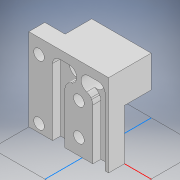
# Autodesk Inventor part: 000.012.001 - Основание
Saved by Autodesk Inventor 2022 (Build 260153000, 153)
## iProperties
Created: 2023-04-23
Part Number: 000.012.001 - Основание
Material: Типовые
Document SubType Name: Modeling
Designer: Иван Петров
Density: 1 g/cm^3
Appearance: По умолчанию
Author: Иван Петров
Autodesk Inventor part; units mm, degrees
ref_plane "YZ Plane" through (0, 0, 0) normal (1, 0, 0) x (0, 1, 0)
ref_plane "XZ Plane" through (0, 0, 0) normal (0, 1, 0) x (-1, 0, 0)
ref_plane "XY Plane" through (0, 0, 0) normal (0, 0, 1) x (1, 0, 0)
sketch "Эскиз1" plane through (0, 0, 0) normal (0, 0, 1) x (1, 0, 0)
  line L0 (-10, -10.5115) -> (10, -10.5115)
  line L1 (10, -10.5115) -> (10, 10.5115)
  line L2 (10, 10.5115) -> (-10, 10.5115)
  line L3 (-10, 10.5115) -> (-10, -10.5115)
  line L4 (-10, -10.5115) -> (10, 10.5115) construction
  line L5 (10, -10.5115) -> (-10, 10.5115) construction
  point P0 (0, 0)
  dimension "d0" = 20
  dimension "d1" = 21.023
  constraints: 12 end point, 2 midpoint, 2 parallel, 1 horizontal, 1 perpendicular
  measures "d0" distance of L2.end L1.end
  measures "d1" distance of L1.end L0.end
extrude "Выдавливание1" add sketch "Эскиз1" along normal blind 6
sketch "Эскиз2" plane through (0, 0, 6) normal (0, 0, 1) x (1, 0, 0)
  circle A0 centre (2.5, 4.5115) radius 2.85 projected
  circle A1 centre (-4.85, 4.5115) radius 2.85 projected
  point P0 (0, 0)
extrude "Выдавливание2" cut sketch "Эскиз2" against normal blind 6
move faces "Перенос1" translate (-10, 0, 0) faces at (-10, 3.5038, 2)
move faces "Перенос2" translate (0, -10, 0) faces at (-10, -10.5115, 2)
sketch "Эскиз4" plane through (0, 0, 0) normal (0, 0, -1) x (-1, 0, 0)
  line L0 (8.6, 0.7615) -> (-3.85, 0.7615) projected
  arc A0 (8.6, 0.7615) -> (9.1, 1.2615) centre (8.6, 1.2615) ccw projected
  line L1 (9.1, 7.7615) -> (9.1, 1.2615) projected
  line L2 (-3.85, 8.2615) -> (8.6, 8.2615) projected
  arc A1 (9.1, 7.7615) -> (8.6, 8.2615) centre (8.6, 7.7615) ccw projected
  line L3 (-6.75, 5.6615) -> (-3.85, 8.2615) projected
  line L4 (-6.75, 3.3615) -> (-6.75, 5.6615) projected
  line L5 (-3.85, 0.7615) -> (-6.75, 3.3615) projected
  line L6 (-10, 10.5115) -> (20, 10.5115) projected
  line L7 (-10, 10.5115) -> (12.35, 10.5115)
  line L8 (12.35, 10.5115) -> (12.35, -1.4885)
  line L9 (12.35, -1.4885) -> (-10, -1.4885)
  line L10 (-10, -1.4885) -> (-10, 10.5115)
  point P0 (0, 0)
  dimension "d19" = 2.25
  dimension "d20" = 2.25
  dimension "d21" = 3.25
  dimension "d23" = 3.25
  constraints: 8 end point, 2 parallel, 1 horizontal, 1 perpendicular
  measures "d19" distance between parallel lines of L6 L2
  measures "d20" distance between parallel lines of L0 L9
  measures "d21" distance between parallel lines of L10 L4
  measures "d23" distance between parallel lines of L8 L1
extrude "Выдавливание4" add sketch "Эскиз4" along normal blind 10
offset faces "Размер1" outward -0.5 faces at (-0.3, 8.2615, -3.3333) (-8.9665, 8.1016, -6.6667) (-9.1, 5.5948, -3.3333) (5.7833, 6.5282, -3.3333) (6.75, 4.1282, -3.3333) (4.8167, 1.6282, -3.3333) (-4.45, 0.7615, -3.3333) (-8.7474, 0.7837, -6.6667)
sketch "Эскиз5" plane through (0, 0, 0) normal (0, 0, -1) x (-1, 0, 0)
  circle A0 centre (16.175, 4.9639) radius 2
  line L0 (12.35, 10.5115) -> (20, 10.5115) projected
  point P0 (0, 0)
  point P1 (16.175, 10.5115)
  dimension "d27" = 4
  constraints: 1 centre point, 1 midpoint, 1 vertical alignment
  measures "d27" diameter of A0
extrude "Выдавливание5" cut sketch "Эскиз5" against normal blind 10
sketch "Эскиз6" plane through (0, 0, 6) normal (0, 0, 1) x (1, 0, 0)
  circle A0 centre (-16.175, -17.4699) radius 2
  circle A1 centre (-16.175, 4.9639) radius 2 projected
  circle A2 centre (-1.1985, -0.3999) radius 2
  point P0 (0, 0)
  dimension "d30" = 4
  dimension "d31" = 4
  constraints: 2 centre point, 1 vertical alignment
  measures "d30" diameter of A0
  measures "d31" diameter of A2
extrude "Выдавливание6" cut sketch "Эскиз6" against normal blind 6.5 contours A0
sketch "Эскиз7" plane through (0, 0, 6) normal (0, 0, 1) x (1, 0, 0)
  circle A0 centre (-4.85, 4.5115) radius 2.85 projected
  line L0 (-4.85, 7.3615) -> (-11.0596, 7.3615)
  line L1 (-11.0596, 7.3615) -> (-11.0596, -20.5115)
  line L2 (-20, -20.5115) -> (10, -20.5115) projected
  line L3 (-5, 1.6655) -> (-6.4302, -0.5077)
  line L4 (-6.4302, -0.5077) -> (-6.4302, -20.5115)
  line L5 (10, 10.5115) -> (-20, 10.5115) projected
  line L6 (-1.175, 10.5115) -> (-1.175, 2.4545) construction
  circle A1 centre (2.5, 4.5115) radius 2.85 projected
  line L7 (-4.85, 4.5115) -> (-4.85, 5.527) construction
  line L8 (2.5, 4.5115) -> (2.5, 5.527) construction
  line L9 (2.5, 7.3615) -> (8.7096, 7.3615)
  line L10 (8.7096, 7.3615) -> (8.7096, -20.5115)
  line L11 (2.65, 1.6655) -> (4.0802, -0.5077)
  line L12 (4.0802, -0.5077) -> (4.0802, -20.5115)
  point P0 (0, 0)
  constraints: 22 end point, 6 symmetric about line, 3 point on line, 3 vertical, 2 perpendicular, 2 point on circle, 1 horizontal, 1 tangent, 1 other
extrude "Выдавливание7" cut sketch "Эскиз7" against normal blind 3 contours A0 L3 L4 L2 L1 L0 | L12 L11 A1 L9 L10 L2
fillet "Сопряжение2" radius 2.75 6 edges at (8.7096, 7.3615, 4.5) (2.65, 1.6655, 4.5) (4.0802, -0.5077, 4.5) (-5, 1.6655, 4.5) (-6.4302, -0.5077, 4.5) (-11.0596, 7.3615, 4.5)
sketch "Эскиз8" plane through (0, 0, 6) normal (0, 0, 1) x (1, 0, 0)
  circle A0 centre (-1.175, -2.5115) radius 2
  circle A1 centre (-1.175, -14.5115) radius 2
  line L0 (-6.4302, -20.5115) -> (4.0802, -20.5115) projected
  circle A2 centre (-1.175, -2.5115) radius 3 construction
  point P0 (0, 0)
  point P1 (-1.175, -20.5115)
  dimension "d39" = 4
  dimension "d40" = 4
  dimension "d41" = 6
  dimension "d42" = 12
  dimension "d43" = 6
  constraints: 3 centre point, 2 vertical alignment, 1 coincident, 1 midpoint
  measures "d39" diameter of A0
  measures "d40" diameter of A1
  measures "d41" distance of point (-1.175, -20.512) A1.centre
  measures "d42" distance of A1.centre A0.centre
  measures "d43" diameter of A2
extrude "Выдавливание8" cut sketch "Эскиз8" against normal up to surface (6 mm away)
equation "\"d20\" = d19"
equation "\"d23\" = d21"
